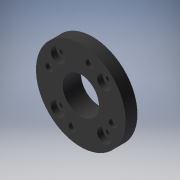
# Autodesk Inventor part: SCHUNK-1013180-ISO-1-50-M6 Universalflansch Co-act-EGP-C
Saved by Autodesk Inventor 2019 (Build 230136000, 136)
## iProperties
Created: 2022-08-29
Part Number: SCHUNK-1013180-ISO-1-50-M6 Universalflansch Co-act-EGP-C
Material: Generic
Catalog Web Link: www.cadenas.de
Description: Flansch Co-act-EGP-C-Co-act EGP-C
Vendor: SCHUNK
Document SubType Name: Modeling
Designer: psAdmin
Manufacturer: SCHUNK
Mass: 25.1643 g
Surface Area: 109.167 cm^2
Volume: 25.1643 cm^3
Density: 1 g/cm^3
Appearance: PSOLRGB-191-191-191
Category: PARTsolutions
Company: SCHUNK
Title: SCHUNK-1013180-ISO-1-50-M6 Universalflansch Co-act-EGP-C
Author: Cadenas PARTsolutions
Comments: Co-act EGP-C
PSOL_IDENT_0: {$CADENAS_DATA/23d-libs/schunk/greifsysteme/greifmodule/co_act/co_act_egp_c/co_act_egp_c_fla.prj},26
PSOL_IDENT_1: 6 {VTYP=3D},{NB=SCHUNK-1013180-ISO-1-50-M6 Universalflansch Co-act-EGP-C},{LINA=SCHUNK-1013180-ISO-1
PSOL_IDENT_2: -50-M6 Universalflansch Co-act-EGP-C},{NN=Flansch Co-act-EGP-C},{DATE=14.05.2021 09:26:35},{GEOMDATE=
PSOL_IDENT_3: 21.04.2021 12:19:14},{VERSION=},{LINEID=20},{WBVAR=},{WBNUMERIC=}  {NB=SCHUNK-1013180-ISO-1-50-M6 Un
PSOL_IDENT_4: iversalflansch Co-act-EGP-C},{LINA=SCHUNK-1013180-ISO-1-50-M6 Universalflansch Co-act-EGP-C},{KT=DUM
PSOL_IDENT_5: MY},{IDNR=1013180},{TYP=ISO-1-50-M6 Universalflansch},{TYP1=2.000},{D1=68.000},{H1=9.100},{H=14.100}
PSOL_IDENT_6: ,{D6=28.000},{D7=31.500},{F1=1.000},{W2=0.600},{TK1=50.000},{TK2=50.000},{W1=15.000},{D2=6.000},{TD2=
PSOL_IDENT_7: 2.900},{D3=4.000},{TGD3=9.100},{TKD3=0.000},{D4=11.000},{TD4=4.600},{D5=6.600},{L1=25.000},{L2=0.500
PSOL_IDENT_8: },{D8=6.000},{TD8=5.500},{D9=0.000},{TD9=0.000},{W3=45.000},{W4=0.000},{T7=0.000},{DY1=0.000},{HY1=0
PSOL_IDENT_9: .000},{HY2=0.000},{RY1=0.000},{RY2=0.000},{WY1=0.000}
NB: SCHUNK-1013180-ISO-1-50-M6 Universalflansch Co-act-EGP-C
NN: Flansch Co-act-EGP-C
NT: Co-act EGP-C
NBSYN: SCHUNK-$IDNR.-$TYP. Co-act-EGP-C
LINA: SCHUNK-1013180-ISO-1-50-M6 Universalflansch Co-act-EGP-C
CATALOG: SCHUNK
IDNR: 1013180
TYP: ISO-1-50-M6 Universalflansch
TYP1: 2
D1: 68
H1: 9.1
H: 14.1
D6: 28
D7: 31.5
F1: 1
W2: 0.6
TK1: 50
TK2: 50
W1: 15
D2: 6
TD2: 2.9
D3: 4
TGD3: 9.1
TKD3: 0
D4: 11
TD4: 4.6
D5: 6.6
L1: 25
L2: 0.5
D8: 6
TD8: 5.5
D9: 0
TD9: 0
W3: 45
W4: 0
T7: 0
DY1: 0
HY1: 0
HY2: 0
RY1: 0
RY2: 0
WY1: 0
SUPPLIER: SCHUNK
ARTICLENO: SCHUNK-1013180-ISO-1-50-M6 Universalflansch Co-act-EGP-C
BOMINFO: SCHUNK-1013180-ISO-1-50-M6 Universalflansch Co-act-EGP-C
CREATOR: CADENAS GmbH
Autodesk Inventor part; units mm, degrees
sketch "Sketch_1" plane through (0, 0, 0) normal (1, 0, 0) x (0, 1, 0)
  line L0 (0, -14.1) -> (0, 0)
  line L1 (34, 0) -> (14, 0)
  line L2 (14, 0) -> (14, -14.1)
  line L3 (14, -14.1) -> (15.75, -14.1)
  line L4 (15.75, -14.1) -> (15.75, -9.1)
  line L5 (15.75, -9.1) -> (34, -9.1)
  line L6 (34, -9.1) -> (34, 0)
  constraints: 14 end point
revolve "Revolution1" add sketch "Sketch_1" angle 360 about axis through (0, 0, -14.1) along (0, 0, 1)
chamfer "Chamfer1" distance 0.6 distance2 1 1 edges at (0, -15.75, -14.1) measured on face at (1.2564, 15.0141, -14.1)
sketch "Sketch2" plane through (0, 0, 0) normal (0, 0, 1) x (1, 0, 0)
  point P0 (24.1481, -6.4705)
hole "Hole1" at (24.1481, -6.4705, 0) direction (0, 0, -1) diameter 3.242 depth 9.1 counterbore diameter 6 counterbore depth 2.9 thread size "M4x0.7" class "6H" standard "ISO Metric profile"
pattern_linear "Rectangular Pattern1" count 2 spacing 35.3553 along (-0.5, 0.866, 0) count 2 spacing 35.3553 along (-0.866, -0.5, 0) of "Hole1"
sketch "Sketch3" plane through (0, 0, 0) normal (0, 0, 1) x (1, 0, 0)
  point P0 (17.6777, -17.6777)
hole "Hole2" at (17.6777, -17.6777, 0) direction (0, 0, -1) diameter 6.6 depth 14.1 counterbore diameter 11 counterbore depth 4.6
pattern_linear "Rectangular Pattern2" count 2 spacing 35.3553 along (0, 1, 0) count 2 spacing 35.3553 along (-1, 0, 0) of "Hole2"
sketch "Sketch_6" plane through (0, 0, -9.1) normal (0, 0, 1) x (1, 0, 0)
  arc A0 (-25.5, 3) -> (-25.5, -3) centre (-25.5, 0) ccw
  line L0 (-25.5, -3) -> (-25, -3)
  arc A1 (-25, -3) -> (-25, 3) centre (-25, 0) ccw
  line L1 (-25, 3) -> (-25.5, 3)
  constraints: 4 end point, 4 point on circle, 2 centre point
extrude "Extrusion1" cut sketch "Sketch_6" along normal blind 5.5
ref_plane "fla_XY" through (0, 0, 0) normal (0, 0, 1) x (1, 0, 0)
ref_plane "fla_YZ" through (0, 0, 0) normal (1, 0, 0) x (0, 1, 0)
ref_plane "fla_ZX" through (0, 0, 0) normal (0, 1, 0) x (0, 0, 1)
body "Solid1"
